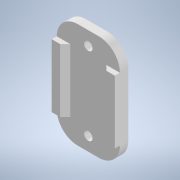
# Autodesk Inventor part: led_cap
Saved by Autodesk Inventor 2022 (Build 260153000, 153)
## iProperties
Created: 2024-07-06
Part Number: led_cap
Material: Типовые
Document SubType Name: Modeling
Designer: Капустяник Андрей
Density: 1 g/cm^3
Appearance: По умолчанию
Author: Капустяник Андрей
Autodesk Inventor part; units mm, degrees
ref_plane "YZ Plane" through (0, 0, 0) normal (1, 0, 0) x (0, 1, 0)
ref_plane "XZ Plane" through (0, 0, 0) normal (0, 1, 0) x (-1, 0, 0)
ref_plane "XY Plane" through (0, 0, 0) normal (0, 0, 1) x (1, 0, 0)
sketch "Эскиз1" plane through (0, 0, 0) normal (0, 0, 1) x (1, 0, 0)
  circle A0 centre (0, 0) radius 6
  line L0 (-7.5, 12.5) -> (7.5, 12.5)
  line L1 (7.5, 12.5) -> (7.5, -12.5)
  line L2 (7.5, -12.5) -> (-7.5, -12.5)
  line L3 (-7.5, -12.5) -> (-7.5, 12.5)
  line L4 (-7.5, 12.5) -> (7.5, -12.5) construction
  line L5 (7.5, 12.5) -> (-7.5, -12.5) construction
  line L6 (0, 6) -> (0, 12.5)
  line L7 (0, -6) -> (0, -12.5)
  circle A1 centre (0, 9.25) radius 1
  circle A2 centre (0, -9.25) radius 1
  dimension "d0" = 12
  dimension "d1" = 15
  dimension "d2" = 25
  dimension "d31" = 2
  dimension "d32" = 2
  constraints: 16 end point, 6 midpoint, 3 centre point, 2 parallel, 2 point on circle, 1 coincident, 1 horizontal, 1 perpendicular, 1 point on line
  measures "d0" diameter of A0
  measures "d1" distance of L1.end L2.end
  measures "d2" distance of L0.end L1.end
  measures "d31" diameter of A1
  measures "d32" diameter of A2
extrude "Выдавливание1" add sketch "Эскиз1" along normal blind 2 contours A0 | A0 L6 A1 L0 L1 L2 L7 A2 | A0 L7 A2 L2 L3 L0 L6 A1
fillet "Сопряжение6" radius 5 4 edges at (-7.5, -12.5, 1) (-7.5, 12.5, 1) (7.5, 12.5, 1) (7.5, -12.5, 1)
sketch "Эскиз7" plane through (0, 0, 2) normal (0, 0, 1) x (1, 0, 0)
  circle A0 centre (0, 0) radius 4
  circle A1 centre (0, 0) radius 6
  line L0 (-7.5, 7.5) -> (-7.5, -7.5) projected
  line L1 (-7.5, 7.5) -> (-5.5, 7.5)
  line L2 (-5.5, 7.5) -> (-5.5, -7.5)
  line L3 (-5.5, -7.5) -> (-7.5, -7.5)
  line L4 (-7.5, -7.5) -> (-7.5, 7.5)
  arc A2 (7.5, 7.5) -> (2.5, 12.5) centre (2.5, 7.5) ccw projected
  line L5 (7.5, 7.5) -> (5.5, 7.5)
  line L6 (5.5, 7.5) -> (5.5, -7.5)
  line L7 (5.5, -7.5) -> (7.5, -7.5)
  line L8 (7.5, -7.5) -> (7.5, 7.5)
  dimension "d34" = 8
  dimension "d35" = 12
  dimension "d36" = 2
  dimension "d37" = 2
  constraints: 16 end point, 4 parallel, 2 centre point, 2 coincident, 2 horizontal, 2 perpendicular, 1 point on line
  measures "d34" diameter of A0
  measures "d35" diameter of A1
  measures "d36" distance of L2.end L3.end
  measures "d37" distance of L7.end L6.end
extrude "Выдавливание7" add sketch "Эскиз7" along normal blind 1.2 contours A1 L6 | A1 L6 L5 L8 L7 | L2 A1 | A1 L2 L3 L0 L1
chamfer "Фаска1" distance 1.2 angle 45 2 edges at (5.5, 0, 2) (-5.5, 0, 2)
